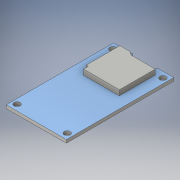
# Autodesk Inventor part: MicroSD Card Reader
Saved by Autodesk Inventor 2016 (Build 200138000, 138)
## iProperties
Created: 2015-11-27
Part Number: MicroSD Card Reader
Material: Generic
Document SubType Name: Modeling
Designer: Spooner
Density: 1 g/cm^3
Appearance: Default
Author: Spooner
Autodesk Inventor part; units mm, degrees
ref_plane "YZ Plane" through (0, 0, 0) normal (1, 0, 0) x (0, 1, 0)
ref_plane "XZ Plane" through (0, 0, 0) normal (0, 1, 0) x (-1, 0, 0)
ref_plane "XY Plane" through (0, 0, 0) normal (0, 0, 1) x (1, 0, 0)
sketch "Sketch1" plane through (0, 0, 0) normal (0, 1, 0) x (-1, 0, 0)
  line L0 (0, 0) -> (-23.5077, 0)
  line L1 (-23.5077, 0) -> (-23.5077, -41.9735)
  line L2 (0, -41.9735) -> (0, 0)
  line L3 (-7.4041, -41.9735) -> (-8.8011, -40.5765)
  line L4 (-8.8011, -40.5765) -> (-16.3322, -40.5765)
  line L5 (-16.3322, -40.5765) -> (-17.7292, -41.9735)
  line L6 (-23.5077, -41.9735) -> (-17.7292, -41.9735)
  line L7 (-7.4041, -41.9735) -> (0, -41.9735)
  circle A0 centre (-1.9431, -39.6748) radius 1.1811
  circle A1 centre (-21.5646, -39.6748) radius 1.1811
  circle A2 centre (-21.5646, -2.2987) radius 1.1811
  circle A3 centre (-1.9431, -2.2987) radius 1.1811
  dimension "d0" = 135
  dimension "d1" = 41.9735
  dimension "d2" = 23.5077
  dimension "d3" = 1.397
  dimension "d4" = 5.7785
  dimension "d5" = 7.4041
  dimension "d6" = 2.3622
  dimension "d7" = 1.1176
  dimension "d8" = 0.762
  dimension "d9" = 0.762
  dimension "d10" = 1.1176
  constraints: 16 end point, 4 centre point, 3 equal radius, 3 horizontal alignment, 3 parallel, 2 horizontal, 2 perpendicular, 2 vertical alignment
  measures "d0" angle of L4 L3
  measures "d1" distance of L2.start L0.start
  measures "d2" distance of L0.start L0.end
  measures "d3" distance between parallel lines of L4 L6
  measures "d4" distance of L1.end L5.end
  measures "d5" distance of L3.start L2.start
  measures "d6" diameter of A0
  measures "d7" distance edge to line of A1 L6
  measures "d8" distance edge to line of A1 L1
  measures "d9" distance edge to line of A0 L2
  measures "d10" distance edge to line of A2 L0
extrude "Extrusion1" add sketch "Sketch1" along normal blind 1.2446
sketch "Sketch2" plane through (0, 1.2446, 0) normal (0, 1, 0) x (1, 0, 0)
  line L0 (9.7028, 39.1795) -> (19.0627, 39.1795)
  line L1 (19.0627, 39.1795) -> (19.0627, 25.146)
  line L2 (19.0627, 25.146) -> (5.08, 25.146)
  line L3 (4.2418, 26.9875) -> (4.2418, 40.1955)
  line L4 (4.2418, 40.1955) -> (8.0518, 40.1955)
  line L5 (8.0518, 40.1955) -> (9.7028, 39.1795)
  line L6 (5.08, 25.146) -> (5.08, 26.9875)
  line L7 (16.3322, 40.5765) -> (8.8011, 40.5765) projected
  line L8 (0, 41.9735) -> (0, 0) projected
  line L9 (4.2418, 26.9875) -> (5.08, 26.9875)
  line L10 (7.4041, 41.9735) -> (0, 41.9735) projected
  point P0 (4.6609, 26.9875)
  dimension "d13" = 14.0335
  dimension "d14" = 1.397
  dimension "d15" = 14.8209
  dimension "d16" = 4.2418
  dimension "d17" = 5.08
  dimension "d18" = 13.208
  dimension "d20" = 1.778
  dimension "d21" = 9.3599
  dimension "d22" = 3.81
  constraints: 16 end point, 2 horizontal, 2 perpendicular, 1 horizontal alignment, 1 midpoint, 1 parallel, 1 vertical
  measures "d13" distance between parallel lines of L2 L0
  measures "d14" distance between parallel lines of L0 L7
  measures "d15" distance between parallel lines of L1 L3
  measures "d16" distance between parallel lines of L8 L3
  measures "d17" distance between parallel lines of L8 L6
  measures "d18" distance of L3.start L3.end
  measures "d20" distance between parallel lines of L4 L10
  measures "d21" distance from line of L0.start L1
  measures "d22" distance of L3.end L4.end
extrude "Extrusion2" add sketch "Sketch2" along normal blind 2.032
sketch "Sketch3" plane through (8.0518, 1.2446, -40.1955) normal (0, 0, -1) x (-1, 0, 0)
  line L0 (-10.1473, 1.778) -> (1.143, 1.778)
  line L1 (1.143, 1.778) -> (1.143, 1.0414)
  line L2 (1.143, 1.0414) -> (-10.1473, 1.0414)
  line L3 (-10.1473, 1.0414) -> (-10.1473, 1.778)
  line L4 (2.9718, 2.032) -> (-11.0109, 2.032) projected
  line L5 (-8.2804, -1.2446) -> (-0.7493, -1.2446) projected
  line L6 (-11.0109, 0) -> (-11.0109, 2.032) projected
  line L7 (3.81, 0) -> (3.81, 2.032) projected
  point P0 (8.0518, -1.2446)
  dimension "d25" = 0.254
  dimension "d26" = 2.286
  dimension "d27" = 0.8636
  dimension "d28" = 2.667
  constraints: 8 end point, 2 parallel, 1 horizontal, 1 perpendicular
  measures "d25" distance between parallel lines of L4 L0
  measures "d26" distance between parallel lines of L5 L2
  measures "d27" distance from line of L6 L0.start
  measures "d28" distance between parallel lines of L7 L1
extrude "Extrusion3" cut sketch "Sketch3" against normal blind 12.192
equation "\"d9\" = d8"
equation "\"d10\" = d7"
body "Solid1"
